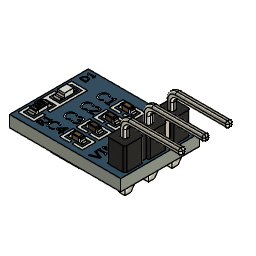
3V (Autodesk Fusion 360 design; units mm, degrees)
Autodesk Fusion 360 part; units mm, degrees
sketch "Sketch1" plane through (0, 0, 0) normal (0, 0, 1) x (1, 0, 0)
  line L0 (6, -4.25) -> (-6, -4.25)
  line L1 (-6, -4.25) -> (-6, 4.25)
  line L2 (-6, 4.25) -> (6, 4.25)
  line L3 (6, 4.25) -> (6, -4.25)
  line L4 (6, -4.25) -> (-6, 4.25) construction
  line L5 (-6, -4.25) -> (6, 4.25) construction
  dimension "d1" = 12
  dimension "d2" = 8.5
  constraint horizontal L0
  constraint perpendicular L0 L1
  constraint parallel L0 L2
  constraint parallel L1 L3
  constraint coincident L4 origin
  constraint coincident L5 origin
  measures "d1" distance of L1.end L2.end
  measures "d2" distance of L0.end L1.end
extrude "Extrude1" add sketch "Sketch1" along normal blind 1.25
sketch "Sketch2" plane through (0, 0, 1.25) normal (0, 0, 1) x (-1, 0, 0)
  line L0 (-6, -4.25) -> (6, -4.25)
  line L1 (6, -4.25) -> (6, 4.25)
  line L2 (6, 4.25) -> (-6, 4.25)
  line L3 (-6, 4.25) -> (-6, -4.25)
  line L4 (-5.75, 3.54) -> (-3.75, 3.54)
  line L5 (-3.75, 3.54) -> (-3.75, 1.54)
  line L6 (-3.75, 1.54) -> (-5.75, 1.54)
  line L7 (-5.75, 1.54) -> (-5.75, 3.54)
  line L8 (-5.75, 3.54) -> (-3.75, 1.54) construction
  line L9 (-3.75, 3.54) -> (-5.75, 1.54) construction
  line L10 (-5.075, 2.865) -> (-4.425, 2.865)
  line L11 (-4.425, 2.865) -> (-4.425, 2.215)
  line L12 (-4.425, 2.215) -> (-5.075, 2.215)
  line L13 (-5.075, 2.215) -> (-5.075, 2.865)
  line L14 (-5.075, 2.865) -> (-4.425, 2.215) construction
  line L15 (-4.425, 2.865) -> (-5.075, 2.215) construction
  line L16 (-5.5, 1.54) -> (-4, 1.54)
  line L17 (-4, 1.54) -> (-4, 1)
  line L18 (-4, 1) -> (-5.5, 1)
  line L19 (-5.5, 1) -> (-5.5, 1.54)
  line L20 (0.75, 2.65) -> (-0.75, 2.65)
  line L21 (-0.75, 2.65) -> (-0.75, 3.15)
  line L22 (-0.75, 3.15) -> (0.75, 3.15)
  line L23 (0.75, 3.15) -> (0.75, 2.65)
  line L24 (0.75, 2.65) -> (-0.75, 3.15) construction
  line L25 (-0.75, 2.65) -> (0.75, 3.15) construction
  line L26 (0.55, 3.15) -> (0.35, 3.15)
  line L27 (0.35, 3.15) -> (0.35, 2.65)
  line L28 (0.35, 2.65) -> (0.55, 2.65)
  line L29 (0.55, 2.65) -> (0.55, 3.15)
  line L30 (-0.35, 3.15) -> (-0.55, 3.15)
  line L31 (-0.55, 3.15) -> (-0.55, 2.65)
  line L32 (-0.55, 2.65) -> (-0.35, 2.65)
  line L33 (-0.35, 2.65) -> (-0.35, 3.15)
  line L34 (5.275, 3.1) -> (4.525, 3.1)
  line L35 (4.525, 3.1) -> (4.525, 1.1)
  line L36 (4.525, 1.1) -> (5.275, 1.1)
  line L37 (5.275, 1.1) -> (5.275, 3.1)
  line L38 (5.275, 3.1) -> (4.525, 1.1) construction
  line L39 (4.525, 3.1) -> (5.275, 1.1) construction
  line L40 (5.275, 1.35) -> (4.525, 1.35)
  line L41 (4.525, 1.35) -> (4.525, 1.6)
  line L42 (4.525, 1.6) -> (5.275, 1.6)
  line L43 (5.275, 1.6) -> (5.275, 1.35)
  line L44 (5.275, 2.6) -> (4.525, 2.6)
  line L45 (4.525, 2.6) -> (4.525, 2.85)
  line L46 (4.525, 2.85) -> (5.275, 2.85)
  line L47 (5.275, 2.85) -> (5.275, 2.6)
  line L48 (0.95, 2.45) -> (-0.95, 2.45)
  line L49 (-0.95, 2.45) -> (-0.95, 3.35)
  line L50 (-0.95, 3.35) -> (0.95, 3.35)
  line L51 (0.95, 3.35) -> (0.95, 2.45)
  line L52 (1.25, 2.15) -> (-1.25, 2.15)
  line L53 (-1.25, 2.15) -> (-1.25, 3.65)
  line L54 (-1.25, 3.65) -> (1.25, 3.65)
  line L55 (1.25, 3.65) -> (1.25, 2.15)
  line L56 (4.325, 0.9) -> (5.475, 0.9)
  line L57 (5.475, 0.9) -> (5.475, 3.3)
  line L58 (5.475, 3.3) -> (4.325, 3.3)
  line L59 (4.325, 3.3) -> (4.325, 0.9)
  line L60 (4.025, 0.6) -> (5.775, 0.6)
  line L61 (5.775, 0.6) -> (5.775, 3.6)
  line L62 (5.775, 3.6) -> (4.025, 3.6)
  line L63 (4.025, 3.6) -> (4.025, 0.6)
  line L64 (0.35, 2.65) -> (-0.35, 2.65)
  line L65 (-0.35, 2.65) -> (-0.35, 2.6501)
  line L66 (-0.35, 2.6501) -> (0.35, 2.6501)
  line L67 (0.35, 2.6501) -> (0.35, 2.65)
  line L68 (-0.35, 3.15) -> (0.35, 3.15)
  line L69 (0.35, 3.15) -> (0.35, 3.1499)
  line L70 (0.35, 3.1499) -> (-0.35, 3.1499)
  line L71 (-0.35, 3.1499) -> (-0.35, 3.15)
  line L72 (0.15, 3.35) -> (-0.15, 3.35)
  line L73 (-0.15, 3.35) -> (-0.15, 3.65)
  line L74 (-0.15, 3.65) -> (0.15, 3.65)
  line L75 (0.15, 3.65) -> (0.15, 3.35)
  line L76 (0.15, 3.35) -> (-0.15, 3.35)
  line L77 (-0.15, 3.35) -> (-0.15, 2.15)
  line L78 (-0.15, 2.15) -> (0.15, 2.15)
  line L79 (0.15, 2.15) -> (0.15, 3.35)
  line L80 (5.275, 2) -> (5.2749, 2)
  line L81 (5.2749, 1.6) -> (5.2749, 2.6)
  line L82 (5.2749, 3) -> (5.275, 3)
  line L83 (5.275, 2.6) -> (5.275, 1.6)
  line L84 (4.525, 1.6) -> (4.5251, 1.6)
  line L85 (4.5251, 1.6) -> (4.5251, 2.6)
  line L86 (4.5251, 2.6) -> (4.525, 2.6)
  line L87 (4.525, 2.6) -> (4.525, 1.6)
  line L88 (5.275, 2) -> (5.2749, 2)
  line L89 (5.2749, 1.6) -> (5.2749, 2.6)
  line L90 (5.2749, 2.6) -> (5.275, 2.6)
  line L91 (5.275, 2.6) -> (5.275, 1.6)
  line L92 (5.475, 1.85) -> (5.775, 1.85)
  line L93 (5.775, 1.85) -> (5.775, 2.35)
  line L94 (5.775, 2.35) -> (5.475, 2.35)
  line L95 (5.475, 2.35) -> (5.475, 1.85)
  line L96 (5.475, 1.85) -> (4.025, 1.85)
  line L97 (4.025, 1.85) -> (4.025, 2.35)
  line L98 (4.025, 2.35) -> (5.475, 2.35)
  line L99 (5.475, 2.35) -> (5.475, 1.85)
  line L100 (5.275, 0.3) -> (4.525, 0.3)
  line L101 (4.525, 0.3) -> (4.525, -1.7)
  line L102 (4.525, -1.7) -> (5.275, -1.7)
  line L103 (5.275, -1.7) -> (5.275, 0.3)
  line L104 (5.275, 0.3) -> (4.525, -1.7) construction
  line L105 (4.525, 0.3) -> (5.275, -1.7) construction
  line L106 (4.525, -1.7) -> (5.275, -1.7)
  line L107 (5.275, -1.7) -> (5.275, -1.2)
  line L108 (5.275, -1.2) -> (4.525, -1.2)
  line L109 (4.525, -1.2) -> (4.525, -1.7)
  line L110 (4.525, 0.3) -> (5.275, 0.3)
  line L111 (5.275, 0.3) -> (5.275, -0.2)
  line L112 (5.275, -0.2) -> (4.525, -0.2)
  line L113 (4.525, -0.2) -> (4.525, 0.3)
  line L114 (4.325, -1.9) -> (5.475, -1.9)
  line L115 (5.475, -1.9) -> (5.475, 0.5)
  line L116 (5.475, 0.5) -> (4.325, 0.5)
  line L117 (4.325, 0.5) -> (4.325, -1.9)
  line L118 (4.025, 0.8) -> (4.025, -2.2)
  line L119 (4.025, -2.2) -> (5.775, -2.2)
  line L120 (5.775, -2.2) -> (5.775, 0.8)
  line L121 (5.775, 0.8) -> (4.025, 0.8)
  line L122 (4.525, -0.2) -> (4.5251, -0.2)
  line L123 (4.5251, -0.2) -> (4.5251, -1.2)
  line L124 (4.5251, -1.2) -> (4.525, -1.2)
  line L125 (4.525, -1.2) -> (4.525, -0.2)
  line L126 (5.275, -0.2) -> (5.2749, -0.2)
  line L127 (5.2749, -0.2) -> (5.2749, -1.2)
  line L128 (5.2749, -1.2) -> (5.275, -1.2)
  line L129 (5.275, -1.2) -> (5.275, -0.2)
  line L130 (5.475, -0.35) -> (5.775, -0.35)
  line L131 (5.775, -0.35) -> (5.775, -0.85)
  line L132 (5.775, -0.85) -> (5.475, -0.85)
  line L133 (5.475, -0.85) -> (5.475, -0.35)
  line L134 (5.475, -0.85) -> (4.025, -0.85)
  line L135 (4.025, -0.85) -> (4.025, -0.35)
  line L136 (4.025, -0.35) -> (5.475, -0.35)
  line L137 (5.475, -0.35) -> (5.475, -0.85)
  point P0 (-4.75, 2.54)
  point P1 (-4.75, 2.54)
  point P2 (0, 2.9)
  point P3 (4.9, 2.1)
  point P4 (4.9, -0.7)
  dimension "d5" = 2
  dimension "d6" = 2
  dimension "d7" = 0.25
  dimension "d8" = 0.71
  dimension "d11" = 0.65
  dimension "d12" = 0.65
  dimension "d28" = 0.54
  dimension "d29" = 0.25
  dimension "d30" = 0.25
  dimension "d35" = 1.5
  dimension "d36" = 0.5
  dimension "d37" = 0.2
  dimension "d38" = 0.2
  dimension "d39" = 0.2
  dimension "d40" = 0.2
  dimension "d41" = 6
  dimension "d52" = 0.75
  dimension "d53" = 2
  dimension "d54" = 0.25
  dimension "d55" = 0.25
  dimension "d56" = 0.25
  dimension "d57" = 0.25
  dimension "d58" = 1.1
  dimension "d59" = 2.15
  dimension "d92" = -0.2
  dimension "d93" = -0.5
  dimension "d96" = 0.2
  dimension "d97" = 0.5
  dimension "d117" = 7.15
  dimension "d118" = 0.0001
  dimension "d119" = 0.0001
  dimension "d120" = 0.3
  dimension "d121" = 1.1
  dimension "d122" = 0.3
  dimension "d123" = 0.0001
  dimension "d124" = 0.0001
  dimension "d125" = 0.0001
  dimension "d128" = 0.5
  dimension "d129" = 1.25
  dimension "d130" = 0.5
  dimension "d131" = 0.75
  dimension "d132" = 2
  dimension "d133" = 1.1
  dimension "d134" = 3.55
  dimension "d135" = 0.5
  dimension "d136" = 0.5
  dimension "d137" = 0.2
  dimension "d138" = 0.5
  dimension "d143" = 0.0001
  dimension "d144" = 0.0001
  dimension "d147" = 0.5
  dimension "d148" = 0.95
  dimension "d149" = 0.5
  constraint horizontal L4
  constraint perpendicular L4 L5
  constraint parallel L4 L6
  constraint parallel L5 L7
  constraint coincident L8 P1
  constraint coincident L9 P1
  constraint horizontal L10
  constraint perpendicular L10 L11
  constraint parallel L10 L12
  constraint parallel L11 L13
  constraint coincident L14 P1
  constraint coincident L15 P1
  constraint coincident P1 P0
  constraint horizontal L16
  constraint vertical L17
  constraint horizontal L18
  constraint vertical L19
  constraint coincident L6 L16.start
  constraint horizontal L20
  constraint perpendicular L20 L21
  constraint parallel L20 L22
  constraint parallel L21 L23
  constraint coincident L24 P2
  constraint coincident L25 P2
  constraint horizontal L26
  constraint vertical L27
  constraint horizontal L28
  constraint vertical L29
  constraint coincident L22 L26.start
  constraint horizontal L30
  constraint vertical L31
  constraint horizontal L32
  constraint vertical L33
  constraint coincident L22 L30.start
  constraint horizontal L34
  constraint perpendicular L34 L35
  constraint parallel L34 L36
  constraint parallel L35 L37
  constraint coincident L38 P3
  constraint coincident L39 P3
  constraint horizontal L40
  constraint vertical L41
  constraint horizontal L42
  constraint vertical L43
  constraint coincident L37 L40.start
  constraint horizontal L44
  constraint vertical L45
  constraint horizontal L46
  constraint vertical L47
  constraint coincident L37 L44.start
  constraint coincident L20 L32.end
  constraint coincident L20 L27.end
  constraint coincident L35 L44.end
  constraint coincident L35 L41.end
  constraint horizontal L64
  constraint vertical L65
  constraint horizontal L66
  constraint vertical L67
  constraint coincident L33 L65.end
  constraint horizontal L68
  constraint vertical L69
  constraint horizontal L70
  constraint vertical L71
  constraint coincident L27 L69.end
  constraint horizontal L72
  constraint vertical L73
  constraint horizontal L74
  constraint vertical L75
  constraint coincident L54 L73.end
  constraint coincident L50 L72.start
  constraint horizontal L76
  constraint vertical L77
  constraint horizontal L78
  constraint vertical L79
  constraint coincident L52 L77.end
  constraint horizontal L80
  constraint vertical L81
  constraint horizontal L82
  constraint vertical L83
  constraint coincident L44 L81.end
  constraint horizontal L84
  constraint vertical L85
  constraint horizontal L86
  constraint vertical L87
  constraint coincident L44 L85.end
  constraint horizontal L88
  constraint vertical L89
  constraint horizontal L90
  constraint vertical L91
  constraint horizontal L92
  constraint vertical L93
  constraint horizontal L94
  constraint vertical L95
  constraint coincident L61 L93.end
  constraint coincident L57 L92.start
  constraint horizontal L96
  constraint vertical L97
  constraint horizontal L98
  constraint vertical L99
  constraint coincident L63 L97.end
  constraint horizontal L100
  constraint perpendicular L100 L101
  constraint parallel L100 L102
  constraint parallel L101 L103
  constraint coincident L104 P4
  constraint coincident L105 P4
  constraint horizontal L106
  constraint vertical L107
  constraint horizontal L108
  constraint vertical L109
  constraint coincident L103 L107.end
  constraint horizontal L110
  constraint vertical L111
  constraint horizontal L112
  constraint vertical L113
  constraint coincident L103 L111.end
  constraint horizontal L122
  constraint vertical L123
  constraint parallel L122 L124
  constraint vertical L125
  constraint horizontal L126
  constraint vertical L127
  constraint parallel L126 L128
  constraint vertical L129
  constraint coincident L108 L127.end
  constraint horizontal L130
  constraint vertical L131
  constraint horizontal L132
  constraint vertical L133
  constraint coincident L120 L131.end
  constraint coincident L115 L130.start
  constraint horizontal L134
  constraint vertical L135
  constraint horizontal L136
  constraint vertical L137
  constraint coincident L118 L135.end
  constraint coincident L108 L123.end
  measures "d5" distance of L5.end L6.end
  measures "d6" distance of L4.end L5.end
  measures "d7" distance of L3 L7
  measures "d8" distance of L2 L4
  measures "d11" distance of L11.end L12.end
  measures "d12" distance of L10.end L11.end
  measures "d28" distance of L16.start L18.end
  measures "d29" distance of L5 L17
  measures "d30" distance of L7 L19
  measures "d35" distance of L21.end L22.end
  measures "d36" distance of L20.end L21.end
  measures "d37" distance of L26.start L26.end
  measures "d38" distance of L30.start L30.end
  measures "d39" distance of L21 L31
  measures "d40" distance of L23 L29
  measures "d41" distance of L3 P2
  measures "d52" distance of L35.end L36.end
  measures "d53" distance of L34.end L35.end
  measures "d54" distance of L40.start L42.end
  measures "d55" distance of L36 L40
  measures "d56" distance of L44.start L46.end
  measures "d57" distance of L34 L46
  measures "d58" distance of L1 P3
  measures "d59" distance of L2 P3
  measures "d117" distance of L0 P2
  measures "d118" distance of L27.end L66.end
  measures "d119" distance of L30.start L70.end
  measures "d120" distance of L72.start L72.end
  measures "d121" distance of L53 L73
  measures "d122" distance of L72.start L72.end
  measures "d123" distance of L42.end L81.start
  measures "d124" distance of L41.end L84.end
  measures "d125" distance of L42.end L81.start
  measures "d128" distance of L92.start L94.end
  measures "d129" distance of L62 L94
  measures "d130" distance of L92.start L94.end
  measures "d131" distance of L101.end L102.end
  measures "d132" distance of L100.end L101.end
  measures "d133" distance of L1 P4
  measures "d134" distance of L0 P4
  measures "d135" distance of L101.end L108.end
  measures "d136" distance of L100.end L112.end
  measures "d143" distance of L112.end L122.end
  measures "d144" distance of L111.end L126.end
  measures "d147" distance of L130.start L132.end
  measures "d148" distance of L60 L130
  measures "d149" distance of L132.end L130.start
extrude "Extrude3" add sketch "Sketch2" along normal blind 4.5 contours L10 L11 L12 L13
extrude "Extrude2" add sketch "Sketch2" along normal blind 2.5 contours L4 L5 L6 L7 L16 | L10 L11 L12 L13
sketch "Sketch3" plane through (5.075, 0, 0) normal (1, 0, 0) x (0, 1, 0)
  line L0 (-2.865, 3.75) -> (-2.215, 3.75)
  line L1 (-2.215, 3.75) -> (-2.215, 5.75)
  line L2 (-2.215, 5.75) -> (-2.865, 5.75)
  line L3 (-2.865, 5.75) -> (-2.865, 3.75)
  line L4 (-2.865, 5.75) -> (-2.215, 5.75)
  line L5 (-2.215, 5.75) -> (-2.215, 5.1)
  line L6 (-2.215, 5.1) -> (-2.865, 5.1)
  line L7 (-2.865, 5.1) -> (-2.865, 5.75)
  dimension "d15" = 0.65
  constraint horizontal L4
  constraint vertical L5
  constraint horizontal L6
  constraint vertical L7
  constraint coincident L2.end L3.start
  constraint coincident L1 L5.end
  measures "d15" distance of L2.end L6.end
extrude "Extrude4" add sketch "Sketch3" along normal blind 6 contours L1 L2 L3 L4 L5 L6 L7
fillet "Fillet1" radius 0.2 16 edges at (5.075, -2.865, 4.425) (4.425, -2.865, 4.75) (5.075, -2.215, 4.425) (4.425, -2.215, 4.75) (7.75, -2.215, 5.75) (8.075, -2.215, 5.1) (7.75, -2.865, 5.75) (11.075, -2.54, 5.75) (11.075, -2.865, 5.425) (11.075, -2.215, 5.425) (11.075, -2.54, 5.1) (8.075, -2.865, 5.1) (5.75, -3.54, 2.5) (3.75, -3.54, 2.5) (5.75, -1.54, 2.5) (3.75, -1.54, 2.5)
fillet "Fillet1" radius 0.5 1 edges at (5.075, -2.54, 5.1)
fillet "Fillet1" radius 1 1 edges at (4.425, -2.54, 5.75)
pattern_linear "R-Pattern1" count 3 spacing 2.54 along (0, 1, 0) of "Extrude3", "Extrude2", "Extrude4", "Fillet1"
extrude "Extrude5" add sketch "Sketch2" along normal blind 2.5 contours L6 L16 L17 L18 L19
mirror "Mirror1" about plane through (0, 0, 0) normal (0, 1, 0) of "Extrude5"
extrude "Extrude6" add sketch "Sketch2" along normal blind 0.5 contours L20 L22 L26 L27 L28 L29 | L20 L22 L30 L31 L32 L33
extrude "Extrude7" add sketch "Sketch2" along normal blind 0.15 contours L20 L22 L23 L29 | L20 L21 L22 L31
extrude "Extrude8" add sketch "Sketch2" along normal blind 0.5001 contours L20 L22 L27 L64 L66 L68 L70 L79 | L20 L22 L64 L66 L68 L70 L77 L79 | L20 L22 L33 L64 L66 L68 L70 L77
fillet "Fillet2" radius 0.15 4 edges at (-0.55, -2.9, 1.4) (-0.75, -2.9, 1.4) (0.55, -2.9, 1.4) (0.75, -2.9, 1.4)
fillet "Fillet2" radius 0.05 8 edges at (0.45, -3.15, 1.75) (0, -3.1499, 1.7501) (-0.45, -3.15, 1.75) (-0.55, -2.9, 1.75) (-0.45, -2.65, 1.75) (0, -2.6501, 1.7501) (0.45, -2.65, 1.75) (0.55, -2.9, 1.75)
extrude "Extrude14" add sketch "Sketch2" along normal blind 0.001 contours L48 L50 L51 L52 L54 L55 L75 L79 | L48 L49 L50 L52 L53 L54 L73 L77
pattern_linear "R-Pattern2" count 4 spacing 1.8 along (0, 1, 0) of "Extrude6", "Extrude7", "Extrude8", "Fillet2", "Extrude14"
extrude "Extrude9" add sketch "Sketch2" along normal blind 0.4 contours L35 L37 L44 L45 L46 L47 | L35 L37 L40 L41 L42 L43
extrude "Extrude10" add sketch "Sketch2" along normal blind 0.15 contours L34 L35 L37 L46 | L35 L36 L37 L40
extrude "Extrude11" add sketch "Sketch2" along normal blind 0.4001 contours L35 L37 L44 L81 L83 L85 L87 L89 L91 L98 | L35 L37 L81 L83 L85 L87 L89 L91 L96 L98 | L35 L37 L42 L81 L83 L85 L87 L89 L91 L96
fillet "Fillet3" radius 0.15 4 edges at (-4.9, -2.85, 1.4) (-4.9, -3.1, 1.4) (-4.9, -1.35, 1.4) (-4.9, -1.1, 1.4)
fillet "Fillet3" radius 0.05 8 edges at (-4.9, -2.85, 1.65) (-5.275, -2.725, 1.65) (-5.2749, -2.1, 1.6501) (-5.275, -1.475, 1.65) (-4.9, -1.35, 1.65) (-4.525, -1.475, 1.65) (-4.5251, -2.1, 1.6501) (-4.525, -2.725, 1.65)
extrude "Extrude15" add sketch "Sketch2" along normal blind 0.001 contours L57 L58 L59 L61 L62 L63 L94 L98 | L56 L57 L59 L61 L63 L92 L96 L121 | L60 L61 L63 L118 L120 L121
extrude "Extrude19" add sketch "Sketch2" along normal blind 0.5 contours L101 L103 L112 L123 L125 L127 L129 L136 | L101 L103 L123 L125 L127 L129 L134 L136 | L101 L103 L108 L123 L125 L127 L129 L134
extrude "Extrude20" add sketch "Sketch2" along normal blind 0.15 contours L100 L101 L103 L110 L111 L112 L113 | L101 L102 L103 L106 L107 L108 L109
fillet "Fillet4" radius 0.15 4 edges at (-4.9, 1.2, 1.4) (-4.9, 1.7, 1.4) (-4.9, 0.2, 1.4) (-4.9, -0.3, 1.4)
extrude "Extrude21" add sketch "Sketch2" along normal blind 0.001 contours L60 L115 L116 L117 L118 L120 L130 L136 | L117 L118 L134 L135 L136 | L114 L115 L117 L118 L119 L120 L132 L134
sketch "Sketch4" plane through (0, 0, 0) normal (0, 0, -1) x (1, 0, 0)
  line L0 (-6, -4.25) -> (6, -4.25)
  line L1 (6, -4.25) -> (6, 4.25)
  line L2 (6, 4.25) -> (-6, 4.25)
  line L3 (-6, 4.25) -> (-6, -4.25)
  circle A0 centre (4.75, 2.54) radius 1
  line L4 (5.075, 2.215) -> (4.425, 2.215)
  line L5 (4.425, 2.215) -> (4.425, 2.865)
  line L6 (4.425, 2.865) -> (5.075, 2.865)
  line L7 (5.075, 2.865) -> (5.075, 2.215)
  line L8 (5.075, 2.215) -> (4.425, 2.865) construction
  line L9 (4.425, 2.215) -> (5.075, 2.865) construction
  point P0 (4.75, 2.54)
  point P1 (4.75, 2.54)
  dimension "d70" = 2
  dimension "d71" = 0.65
  dimension "d72" = 0.65
  constraint coincident P1 P0
  constraint horizontal L4
  constraint perpendicular L4 L5
  constraint parallel L4 L6
  constraint parallel L5 L7
  constraint coincident L8 P1
  constraint coincident L9 P1
  measures "d70" diameter of A0
  measures "d71" distance of L5.end L6.end
  measures "d72" distance of L4.end L5.end
extrude "Extrude12" add sketch "Sketch4" along normal blind 1.5 contours L4 L5 L6 L7
loft "Loft1" add profiles "Sketch4" section 1 contours A0 section 2 face at (4.8583, -2.4317, -1.5)
pattern_linear "R-Pattern4" count 3 spacing 2.54 along (0, 1, 0) of "Extrude12", "Loft1"
sketch "Sketch5" plane through (0, 0, 0) normal (0, 0, -1) x (1, 0, 0)
  spline S0 degree 3 poles (4.0429, -1.8329) (4.2258, -1.65) (4.4818, -1.5425) (4.7404, -1.54) (5.0054, -1.5375) (5.2697, -1.6455) (5.4571, -1.8329) knots -1 -1 -1 -1 -0.506107 -0.506107 -0.506107 0 0 0 0
  spline S1 degree 3 poles (5.4571, -1.8329) (5.64, -2.0158) (5.7475, -2.2718) (5.75, -2.5304) (5.7525, -2.7954) (5.6445, -3.0597) (5.4571, -3.2471) knots -1 -1 -1 -1 -0.506107 -0.506107 -0.506107 0 0 0 0
  spline S2 degree 3 poles (5.4571, -3.2471) (5.2742, -3.43) (5.0182, -3.5375) (4.7596, -3.54) (4.4946, -3.5425) (4.2303, -3.4345) (4.0429, -3.2471) knots -1 -1 -1 -1 -0.506107 -0.506107 -0.506107 0 0 0 0
  spline S3 degree 3 poles (4.0429, -3.2471) (3.86, -3.0642) (3.7525, -2.8082) (3.75, -2.5496) (3.7475, -2.2846) (3.8555, -2.0203) (4.0429, -1.8329) knots -1 -1 -1 -1 -0.506107 -0.506107 -0.506107 0 0 0 0
  spline S4 degree 3 poles (4.0429, 0.7071) (4.2258, 0.89) (4.4818, 0.9975) (4.7404, 1) (5.0054, 1.0025) (5.2697, 0.8945) (5.4571, 0.7071) knots -1 -1 -1 -1 -0.506107 -0.506107 -0.506107 0 0 0 0
  spline S5 degree 3 poles (5.4571, 0.7071) (5.64, 0.5242) (5.7475, 0.2682) (5.75, 0.0096) (5.7525, -0.2554) (5.6445, -0.5197) (5.4571, -0.7071) knots -1 -1 -1 -1 -0.506107 -0.506107 -0.506107 0 0 0 0
  spline S6 degree 3 poles (5.4571, -0.7071) (5.2742, -0.89) (5.0182, -0.9975) (4.7596, -1) (4.4946, -1.0025) (4.2303, -0.8945) (4.0429, -0.7071) knots -1 -1 -1 -1 -0.506107 -0.506107 -0.506107 0 0 0 0
  spline S7 degree 3 poles (4.0429, -0.7071) (3.86, -0.5242) (3.7525, -0.2682) (3.75, -0.0096) (3.7475, 0.2554) (3.8555, 0.5197) (4.0429, 0.7071) knots -1 -1 -1 -1 -0.506107 -0.506107 -0.506107 0 0 0 0
  spline S8 degree 3 poles (4.0429, 3.2471) (4.2258, 3.43) (4.4818, 3.5375) (4.7404, 3.54) (5.0054, 3.5425) (5.2697, 3.4345) (5.4571, 3.2471) knots -1 -1 -1 -1 -0.506107 -0.506107 -0.506107 0 0 0 0
  spline S9 degree 3 poles (5.4571, 3.2471) (5.64, 3.0642) (5.7475, 2.8082) (5.75, 2.5496) (5.7525, 2.2846) (5.6445, 2.0203) (5.4571, 1.8329) knots -1 -1 -1 -1 -0.506107 -0.506107 -0.506107 0 0 0 0
  spline S10 degree 3 poles (5.4571, 1.8329) (5.2742, 1.65) (5.0182, 1.5425) (4.7596, 1.54) (4.4946, 1.5375) (4.2303, 1.6455) (4.0429, 1.8329) knots -1 -1 -1 -1 -0.506107 -0.506107 -0.506107 0 0 0 0
  spline S11 degree 3 poles (4.0429, 1.8329) (3.86, 2.0158) (3.7525, 2.2718) (3.75, 2.5304) (3.7475, 2.7954) (3.8555, 3.0597) (4.0429, 3.2471) knots -1 -1 -1 -1 -0.506107 -0.506107 -0.506107 0 0 0 0
  line L0 (-6, -4.25) -> (6, -4.25)
  line L1 (6, -4.25) -> (6, 4.25)
  line L2 (6, 4.25) -> (-6, 4.25)
  line L3 (-6, 4.25) -> (-6, -4.25)
  line L4 (0.25, -3) -> (-3.25, -3)
  line L5 (-3.25, -3) -> (-3.25, 3)
  line L6 (-3.25, 3) -> (0.25, 3)
  line L7 (0.25, 3) -> (0.25, -3)
  line L8 (0.25, -3) -> (-3.25, 3) construction
  line L9 (-3.25, -3) -> (0.25, 3) construction
  point P0 (-1.5, 0)
  dimension "d152" = 3.5
  dimension "d153" = 6
  dimension "d154" = 4.5
  dimension "d155" = 4.25
  constraint horizontal L4
  constraint perpendicular L4 L5
  constraint parallel L4 L6
  constraint parallel L5 L7
  constraint coincident L8 P0
  constraint coincident L9 P0
  measures "d152" distance of L5.end L6.end
  measures "d153" distance of L4.end L5.end
  measures "d154" distance of L3 P0
  measures "d155" distance of L2 P0
extrude "Extrude22" add sketch "Sketch5" along normal blind 1.5 contours L4 L5 L6 L7
chamfer "Chamfer2" distance 0.2 distance2 0.9 1 faces at (-0.9167, 1, -1.5)
sketch "Sketch6" plane through (-3.25, 0, 0) normal (-1, 0, 0) x (0, -1, 0)
  line L0 (-3, -0.6) -> (3, -0.6)
  line L1 (3, -0.6) -> (3, 0)
  line L2 (3, 0) -> (-3, 0)
  line L3 (-3, 0) -> (-3, -0.6)
  line L4 (1.5, -0.6) -> (-1.5, -0.6)
  line L5 (-1.5, -0.6) -> (-1.5, -0.45)
  line L6 (-1.5, -0.45) -> (1.5, -0.45)
  line L7 (1.5, -0.45) -> (1.5, -0.6)
  dimension "d160" = 3
  dimension "d161" = 0.15
  dimension "d162" = 1.5
  constraint horizontal L4
  constraint vertical L5
  constraint horizontal L6
  constraint vertical L7
  constraint coincident L0 L4.start
  measures "d160" distance of L4.start L4.end
  measures "d161" distance of L4.start L6.end
  measures "d162" distance of L3 L5
extrude "Extrude23" add sketch "Sketch6" along normal blind 0.7 contours L0 L4 L5 L6 L7
sketch "Sketch7" plane through (0, 0, -0.6) normal (0, 0, -1) x (1, 0, 0)
  line L0 (-3.25, -1.5) -> (-3.25, 1.5)
  line L1 (-3.25, 1.5) -> (-3.95, 1.5)
  line L2 (-3.95, 1.5) -> (-3.95, -1.5)
  line L3 (-3.95, -1.5) -> (-3.25, -1.5)
  line L4 (-3.95, -1.5) -> (-3.8, -1.5)
  line L5 (-3.8, -1.5) -> (-3.8, 1.5)
  line L6 (-3.8, 1.5) -> (-3.95, 1.5)
  line L7 (-3.95, 1.5) -> (-3.95, -1.5)
  dimension "d165" = 0.15
  dimension "d166" = 3
  constraint horizontal L4
  constraint vertical L5
  constraint horizontal L6
  constraint vertical L7
  constraint coincident L2.end L3.start
  measures "d165" distance of L2.end L4.end
  measures "d166" distance of L2.end L1.end
extrude "Extrude24" add sketch "Sketch7" against normal blind 0.7 contours L1 L2 L3 L4 L5 L6 L7
sketch "Sketch8" plane through (-3.95, 0, 0) normal (-1, 0, 0) x (0, -1, 0)
  line L0 (-1.5, 0) -> (-1.5, -0.6)
  line L1 (-1.5, -0.6) -> (1.5, -0.6)
  line L2 (1.5, -0.6) -> (1.5, 0)
  line L3 (1.5, 0) -> (-1.5, 0)
  line L4 (1.5, 0) -> (-1.5, 0)
  line L5 (-1.5, 0) -> (-1.5, -0.15)
  line L6 (-1.5, -0.15) -> (1.5, -0.15)
  line L7 (1.5, -0.15) -> (1.5, 0)
  dimension "d169" = 0.15
  constraint horizontal L4
  constraint vertical L5
  constraint horizontal L6
  constraint vertical L7
  constraint coincident L0 L5.end
  constraint coincident L2.end L3.start
  measures "d169" distance of L2.end L6.end
extrude "Extrude25" add sketch "Sketch8" along normal blind 0.5 contours L0 L2 L3 L4 L5 L6 L7
fillet "Fillet5" radius 0.15 4 edges at (-3.95, 0, -0.6) (-3.95, 0, -0.15) (-4.45, 0, -0.15) (-3.8, 0, -0.45)
sketch "Sketch9" plane through (0, -1.5, 0) normal (0, -1, 0) x (1, 0, 0)
  arc A0 (-4.45, 0) -> (-4.3, -0.15) centre (-4.3, 0) ccw
  line L0 (-4.3, -0.15) -> (-4.1, -0.15)
  arc A1 (-3.95, -0.3) -> (-4.1, -0.15) centre (-4.1, -0.3) ccw
  line L1 (-3.95, -0.3) -> (-3.95, -0.45)
  arc A2 (-3.95, -0.45) -> (-3.8, -0.6) centre (-3.8, -0.45) ccw
  line L2 (-3.8, -0.6) -> (-3.25, -0.6)
  line L3 (-3.25, -0.6) -> (-3.25, -0.45)
  line L4 (-3.25, -0.45) -> (-3.65, -0.45)
  arc A3 (-3.8, -0.3) -> (-3.65, -0.45) centre (-3.65, -0.3) ccw
  line L5 (-3.8, -0.3) -> (-3.8, 0)
  line L6 (-3.8, 0) -> (-4.45, 0)
  line L7 (-4.45, 0) -> (-4.1, 0)
  arc A4 (-3.8, -0.3) -> (-4.1, 0) centre (-4.1, -0.3) ccw
  line L8 (-3.8, -0.3) -> (-3.8, -0.45)
  line L9 (-3.8, -0.45) -> (-3.25, -0.45)
  dimension "d174" = -0.15
  constraint coincident L3 L4.start
  constraint coincident A0.start L6.end
extrude "Extrude26" cut sketch "Sketch9" against normal blind 3 contours L5 L6 A4
sketch "Sketch10" plane through (0.25, 0, 0) normal (1, 0, 0) x (0, 1, 0)
  line L0 (-3, -0.6) -> (3, -0.6)
  line L1 (3, -0.6) -> (3, 0)
  line L2 (3, 0) -> (-3, 0)
  line L3 (-3, 0) -> (-3, -0.6)
  line L4 (2.75, -0.6) -> (1.75, -0.6)
  line L5 (1.75, -0.6) -> (1.75, -0.45)
  line L6 (1.75, -0.45) -> (2.75, -0.45)
  line L7 (2.75, -0.45) -> (2.75, -0.6)
  dimension "d177" = 1
  dimension "d178" = 0.15
  dimension "d179" = 0.25
  constraint horizontal L4
  constraint vertical L5
  constraint horizontal L6
  constraint vertical L7
  constraint coincident L0 L4.start
  measures "d177" distance of L4.start L4.end
  measures "d178" distance of L4.start L6.end
  measures "d179" distance of L1 L7
extrude "Extrude27" add sketch "Sketch10" along normal blind 0.7 contours L0 L4 L5 L6 L7
sketch "Sketch11" plane through (0, 0, -0.6) normal (0, 0, -1) x (1, 0, 0)
  line L0 (0.25, -1.75) -> (0.25, -2.75)
  line L1 (0.25, -2.75) -> (0.95, -2.75)
  line L2 (0.95, -2.75) -> (0.95, -1.75)
  line L3 (0.95, -1.75) -> (0.25, -1.75)
  line L4 (0.95, -1.75) -> (0.8, -1.75)
  line L5 (0.8, -1.75) -> (0.8, -2.75)
  line L6 (0.8, -2.75) -> (0.95, -2.75)
  line L7 (0.95, -2.75) -> (0.95, -1.75)
  dimension "d182" = 0.15
  constraint horizontal L4
  constraint vertical L5
  constraint horizontal L6
  constraint vertical L7
  constraint coincident L1 L5.end
  constraint coincident L2.end L3.start
  measures "d182" distance of L2.end L4.end
extrude "Extrude28" add sketch "Sketch11" against normal blind 0.7 contours L1 L2 L3 L4 L5 L6 L7
sketch "Sketch12" plane through (0.95, 0, 0) normal (1, 0, 0) x (0, 1, 0)
  line L0 (1.75, 0) -> (1.75, -0.6)
  line L1 (1.75, -0.6) -> (2.75, -0.6)
  line L2 (2.75, -0.6) -> (2.75, 0)
  line L3 (2.75, 0) -> (1.75, 0)
  line L4 (2.75, 0) -> (1.75, 0)
  line L5 (1.75, 0) -> (1.75, -0.15)
  line L6 (1.75, -0.15) -> (2.75, -0.15)
  line L7 (2.75, -0.15) -> (2.75, 0)
  dimension "d185" = 0.15
  constraint horizontal L4
  constraint vertical L5
  constraint horizontal L6
  constraint vertical L7
  constraint coincident L0 L5.end
  constraint coincident L2.end L3.start
  measures "d185" distance of L2.end L6.end
extrude "Extrude29" add sketch "Sketch12" along normal blind 0.5 contours L0 L2 L3 L4 L5 L6 L7
fillet "Fillet6" radius 0.15 4 edges at (0.95, 2.25, -0.6) (0.95, 2.25, -0.15) (1.45, 2.25, -0.15) (0.8, 2.25, -0.45)
sketch "Sketch13" plane through (0, 2.75, 0) normal (0, 1, 0) x (-1, 0, 0)
  arc A0 (-1.45, 0) -> (-1.3, -0.15) centre (-1.3, 0) ccw
  line L0 (-1.3, -0.15) -> (-1.1, -0.15)
  arc A1 (-0.95, -0.3) -> (-1.1, -0.15) centre (-1.1, -0.3) ccw
  line L1 (-0.95, -0.3) -> (-0.95, -0.45)
  arc A2 (-0.95, -0.45) -> (-0.8, -0.6) centre (-0.8, -0.45) ccw
  line L2 (-0.8, -0.6) -> (-0.25, -0.6)
  line L3 (-0.25, -0.6) -> (-0.25, -0.45)
  line L4 (-0.25, -0.45) -> (-0.65, -0.45)
  arc A3 (-0.8, -0.3) -> (-0.65, -0.45) centre (-0.65, -0.3) ccw
  line L5 (-0.8, -0.3) -> (-0.8, 0)
  line L6 (-0.8, 0) -> (-1.45, 0)
  line L7 (-1.45, 0) -> (-1.1, 0)
  arc A4 (-0.8, -0.3) -> (-1.1, 0) centre (-1.1, -0.3) ccw
  line L8 (-0.8, -0.3) -> (-0.8, -0.45)
  line L9 (-0.8, -0.45) -> (-0.25, -0.45)
  dimension "d190" = -0.15
  constraint coincident A0.start L6.end
  constraint coincident L3 L4.start
extrude "Extrude30" cut sketch "Sketch13" against normal blind 1 contours L5 L6 A4
pattern_linear "R-Pattern5" count 3 spacing 2.25 along (0, -1, 0) of "Extrude27", "Extrude28", "Extrude29", "Fillet6", "Extrude30"
sketch "Sketch14" plane through (0, 0, 1.25) normal (0, 0, 1) x (-1, 0, 0)
  line L0 (-6, -4.25) -> (6, -4.25)
  line L1 (6, -4.25) -> (6, 4.25)
  line L2 (6, 4.25) -> (-6, 4.25)
  line L3 (-6, 4.25) -> (-6, -4.25)
  line L4 (-5.5, -1.54) -> (-5.5, -1)
  line L5 (-5.5, -1) -> (-5.55, -1)
  arc A0 (-5.75, -0.8) -> (-5.55, -1) centre (-5.55, -0.8) ccw
  line L6 (-5.75, -0.8) -> (-5.75, 0.8)
  arc A1 (-5.55, 1) -> (-5.75, 0.8) centre (-5.55, 0.8) ccw
  line L7 (-5.55, 1) -> (-5.5, 1)
  line L8 (-5.5, 1) -> (-5.5, 1.54)
  line L9 (-5.5, 1.54) -> (-5.55, 1.54)
  arc A2 (-5.75, 1.74) -> (-5.55, 1.54) centre (-5.55, 1.74) ccw
  line L10 (-5.75, 1.74) -> (-5.75, 3.34)
  arc A3 (-5.55, 3.54) -> (-5.75, 3.34) centre (-5.55, 3.34) ccw
  line L11 (-5.55, 3.54) -> (-3.95, 3.54)
  arc A4 (-3.75, 3.34) -> (-3.95, 3.54) centre (-3.95, 3.34) ccw
  line L12 (-3.75, 3.34) -> (-3.75, 1.74)
  arc A5 (-3.95, 1.54) -> (-3.75, 1.74) centre (-3.95, 1.74) ccw
  line L13 (-3.95, 1.54) -> (-4, 1.54)
  line L14 (-4, 1.54) -> (-4, 1)
  line L15 (-4, 1) -> (-3.95, 1)
  arc A6 (-3.75, 0.8) -> (-3.95, 1) centre (-3.95, 0.8) ccw
  line L16 (-3.75, 0.8) -> (-3.75, -0.8)
  arc A7 (-3.95, -1) -> (-3.75, -0.8) centre (-3.95, -0.8) ccw
  line L17 (-3.95, -1) -> (-4, -1)
  line L18 (-4, -1) -> (-4, -1.54)
  line L19 (-4, -1.54) -> (-3.95, -1.54)
  arc A8 (-3.75, -1.74) -> (-3.95, -1.54) centre (-3.95, -1.74) ccw
  line L20 (-3.75, -1.74) -> (-3.75, -3.34)
  arc A9 (-3.95, -3.54) -> (-3.75, -3.34) centre (-3.95, -3.34) ccw
  line L21 (-3.95, -3.54) -> (-5.55, -3.54)
  arc A10 (-5.75, -3.34) -> (-5.55, -3.54) centre (-5.55, -3.34) ccw
  line L22 (-5.75, -3.34) -> (-5.75, -1.74)
  arc A11 (-5.55, -1.54) -> (-5.75, -1.74) centre (-5.55, -1.74) ccw
  line L23 (-5.55, -1.54) -> (-5.5, -1.54)
  line L24 (1.25, 3.65) -> (1.25, 2.15)
  line L25 (-0.15, 2.15) -> (-1.25, 2.15)
  line L26 (-1.25, 2.15) -> (-1.25, 3.65)
  line L27 (-1.25, 3.65) -> (-0.15, 3.65)
  line L28 (1.25, 1.85) -> (1.25, 0.35)
  line L29 (1.25, 0.35) -> (0.15, 0.35)
  line L30 (-1.25, 0.35) -> (-1.25, 1.85)
  line L31 (0.15, 1.85) -> (1.25, 1.85)
  line L32 (1.25, 0.05) -> (1.25, -1.45)
  line L33 (-0.15, -1.45) -> (-1.25, -1.45)
  line L34 (-1.25, -1.45) -> (-1.25, 0.05)
  line L35 (-1.25, 0.05) -> (-0.15, 0.05)
  line L36 (1.25, -1.75) -> (1.25, -3.25)
  line L37 (1.25, -3.25) -> (0.15, -3.25)
  line L38 (-1.25, -3.25) -> (-1.25, -1.75)
  line L39 (0.15, -1.75) -> (1.25, -1.75)
  line L40 (4.025, 3.6) -> (5.775, 3.6)
  line L41 (5.775, 1.85) -> (5.775, -0.35)
  line L42 (4.025, -2.2) -> (4.025, 1.85)
  line L43 (3.1789, -1.7897) -> (1.3303, -1.7897) construction
  line L44 (1.3303, -1.7897) -> (1.3303, -3.1651) construction
  line L45 (1.3303, -3.1651) -> (3.1789, -3.1651) construction
  line L46 (3.1789, -3.1651) -> (3.1789, -1.7897) construction
  line L47 (3.1855, -0.0301) -> (1.3369, -0.0301) construction
  line L48 (1.3369, -0.0301) -> (1.3369, -1.4054) construction
  line L49 (1.3369, -1.4054) -> (3.1855, -1.4054) construction
  line L50 (3.1855, -1.4054) -> (3.1855, -0.0301) construction
  line L51 (3.1525, 3.5727) -> (1.3038, 3.5727) construction
  line L52 (1.3038, 3.5727) -> (1.3038, 2.1974) construction
  line L53 (1.3038, 2.1974) -> (3.1525, 2.1974) construction
  line L54 (3.1525, 2.1974) -> (3.1525, 3.5727) construction
  line L55 (3.1627, 1.7821) -> (1.3141, 1.7821) construction
  line L56 (1.3141, 1.7821) -> (1.3141, 0.4068) construction
  line L57 (1.3141, 0.4068) -> (3.1627, 0.4068) construction
  line L58 (3.1627, 0.4068) -> (3.1627, 1.7821) construction
  line L59 (-3.209, 3.6614) -> (-3.209, 1.8128) construction
  line L60 (-3.209, 1.8128) -> (-1.8337, 1.8128) construction
  line L61 (-1.8337, 1.8128) -> (-1.8337, 3.6614) construction
  line L62 (-1.8337, 3.6614) -> (-3.209, 3.6614) construction
  line L63 (-3.209, 1.0614) -> (-3.209, -0.7872) construction
  line L64 (-3.209, -0.7872) -> (-1.8337, -0.7872) construction
  line L65 (-1.8337, -0.7872) -> (-1.8337, 1.0614) construction
  line L66 (-1.8337, 1.0614) -> (-3.209, 1.0614) construction
  line L67 (-3.209, -1.6886) -> (-3.209, -3.5372) construction
  line L68 (-3.209, -3.5372) -> (-1.8337, -3.5372) construction
  line L69 (-1.8337, -3.5372) -> (-1.8337, -1.6886) construction
  line L70 (-1.8337, -1.6886) -> (-3.209, -1.6886) construction
  line L71 (2.8382, 3.8814) -> (2.8382, 2.0328) construction
  line L72 (2.8382, 2.0328) -> (4.2136, 2.0328) construction
  line L73 (4.2136, 2.0328) -> (4.2136, 3.8814) construction
  line L74 (4.2136, 3.8814) -> (2.8382, 3.8814) construction
  line L75 (4.5641, -2.5206) -> (4.5641, -4.3692) construction
  line L76 (4.5641, -4.3692) -> (5.9395, -4.3692) construction
  line L77 (5.9395, -4.3692) -> (5.9395, -2.5206) construction
  line L78 (5.9395, -2.5206) -> (4.5641, -2.5206) construction
  line L79 (4.025, 1.85) -> (4.325, 1.85)
  line L80 (4.325, 1.85) -> (4.325, 0.9)
  line L81 (4.325, 0.9) -> (5.475, 0.9)
  line L82 (5.475, 0.9) -> (5.475, 1.85)
  line L83 (5.475, 1.85) -> (5.775, 1.85)
  line L84 (5.775, -0.35) -> (5.475, -0.35)
  line L85 (5.475, -0.35) -> (5.475, 0.5)
  line L86 (5.475, 0.5) -> (4.325, 0.5)
  line L87 (4.325, 0.5) -> (4.325, -1.9)
  line L88 (4.325, -1.9) -> (5.475, -1.9)
  line L89 (5.475, -1.9) -> (5.475, -0.85)
  line L90 (5.475, -0.85) -> (5.775, -0.85)
  line L91 (5.775, -0.85) -> (5.775, -2.2)
  line L92 (5.775, -2.2) -> (4.025, -2.2)
  line L93 (0.15, -3.25) -> (0.15, -2.95)
  line L94 (0.15, -2.95) -> (0.95, -2.95)
  line L95 (0.95, -2.95) -> (0.95, -2.05)
  line L96 (0.95, -2.05) -> (0.15, -2.05)
  line L97 (0.15, -2.05) -> (0.15, -1.75)
  line L98 (-0.15, -3.25) -> (-1.25, -3.25)
  line L99 (-1.25, -1.75) -> (-0.15, -1.75)
  line L100 (-0.15, -1.75) -> (-0.15, -2.05)
  line L101 (-0.15, -2.05) -> (-0.95, -2.05)
  line L102 (-0.95, -2.05) -> (-0.95, -2.95)
  line L103 (-0.95, -2.95) -> (-0.15, -2.95)
  line L104 (-0.15, -2.95) -> (-0.15, -3.25)
  line L105 (0.35, -0.9499) -> (-0.35, -0.9499)
  line L106 (-0.35, -0.9499) -> (-0.35, -0.95)
  line L107 (-0.35, -0.95) -> (-0.75, -0.95)
  line L108 (-0.75, -0.95) -> (-0.75, -0.45)
  line L109 (-0.75, -0.45) -> (-0.35, -0.45)
  line L110 (-0.35, -0.45) -> (-0.35, -0.4501)
  line L111 (-0.35, -0.4501) -> (0.35, -0.4501)
  line L112 (0.35, -0.4501) -> (0.35, -0.45)
  line L113 (0.35, -0.45) -> (0.75, -0.45)
  line L114 (0.75, -0.45) -> (0.75, -0.95)
  line L115 (0.75, -0.95) -> (0.35, -0.95)
  line L116 (0.35, -0.95) -> (0.35, -0.9499)
  line L117 (0.15, 0.35) -> (0.15, 0.65)
  line L118 (0.15, 0.65) -> (0.95, 0.65)
  line L119 (0.95, 0.65) -> (0.95, 1.55)
  line L120 (0.95, 1.55) -> (0.15, 1.55)
  line L121 (0.15, 1.55) -> (0.15, 1.85)
  line L122 (-0.15, 0.35) -> (-1.25, 0.35)
  line L123 (-1.25, 1.85) -> (-0.15, 1.85)
  line L124 (-0.15, 1.85) -> (-0.15, 1.55)
  line L125 (-0.15, 1.55) -> (-0.95, 1.55)
  line L126 (-0.95, 1.55) -> (-0.95, 0.65)
  line L127 (-0.95, 0.65) -> (-0.15, 0.65)
  line L128 (-0.15, 0.65) -> (-0.15, 0.35)
  line L129 (0.35, 2.6501) -> (-0.35, 2.6501)
  line L130 (-0.35, 2.6501) -> (-0.35, 2.65)
  line L131 (-0.35, 2.65) -> (-0.75, 2.65)
  line L132 (-0.75, 2.65) -> (-0.75, 3.15)
  line L133 (-0.75, 3.15) -> (-0.35, 3.15)
  line L134 (-0.35, 3.15) -> (-0.35, 3.1499)
  line L135 (-0.35, 3.1499) -> (0.35, 3.1499)
  line L136 (0.35, 3.1499) -> (0.35, 3.15)
  line L137 (0.35, 3.15) -> (0.75, 3.15)
  line L138 (0.75, 3.15) -> (0.75, 2.65)
  line L139 (0.75, 2.65) -> (0.35, 2.65)
  line L140 (0.35, 2.65) -> (0.35, 2.6501)
  line L141 (-0.15, 3.65) -> (-0.15, 3.35)
  line L142 (-0.15, 3.35) -> (-0.95, 3.35)
  line L143 (-0.95, 3.35) -> (-0.95, 2.45)
  line L144 (-0.95, 2.45) -> (-0.15, 2.45)
  line L145 (-0.15, 2.45) -> (-0.15, 2.15)
  line L146 (0.15, 3.65) -> (1.25, 3.65)
  line L147 (1.25, 2.15) -> (0.15, 2.15)
  line L148 (0.15, 2.15) -> (0.15, 2.45)
  line L149 (0.15, 2.45) -> (0.95, 2.45)
  line L150 (0.95, 2.45) -> (0.95, 3.35)
  line L151 (0.95, 3.35) -> (0.15, 3.35)
  line L152 (0.15, 3.35) -> (0.15, 3.65)
  line L153 (0.35, 0.8501) -> (-0.35, 0.8501)
  line L154 (-0.35, 0.8501) -> (-0.35, 0.85)
  line L155 (-0.35, 0.85) -> (-0.75, 0.85)
  line L156 (-0.75, 0.85) -> (-0.75, 1.35)
  line L157 (-0.75, 1.35) -> (-0.35, 1.35)
  line L158 (-0.35, 1.35) -> (-0.35, 1.3499)
  line L159 (-0.35, 1.3499) -> (0.35, 1.3499)
  line L160 (0.35, 1.3499) -> (0.35, 1.35)
  line L161 (0.35, 1.35) -> (0.75, 1.35)
  line L162 (0.75, 1.35) -> (0.75, 0.85)
  line L163 (0.75, 0.85) -> (0.35, 0.85)
  line L164 (0.35, 0.85) -> (0.35, 0.8501)
  line L165 (-0.15, 0.05) -> (-0.15, -0.25)
  line L166 (-0.15, -0.25) -> (-0.95, -0.25)
  line L167 (-0.95, -0.25) -> (-0.95, -1.15)
  line L168 (-0.95, -1.15) -> (-0.15, -1.15)
  line L169 (-0.15, -1.15) -> (-0.15, -1.45)
  line L170 (0.15, 0.05) -> (1.25, 0.05)
  line L171 (1.25, -1.45) -> (0.15, -1.45)
  line L172 (0.15, -1.45) -> (0.15, -1.15)
  line L173 (0.15, -1.15) -> (0.95, -1.15)
  line L174 (0.95, -1.15) -> (0.95, -0.25)
  line L175 (0.95, -0.25) -> (0.15, -0.25)
  line L176 (0.15, -0.25) -> (0.15, 0.05)
  line L177 (0.35, -2.7499) -> (-0.35, -2.7499)
  line L178 (-0.35, -2.7499) -> (-0.35, -2.75)
  line L179 (-0.35, -2.75) -> (-0.75, -2.75)
  line L180 (-0.75, -2.75) -> (-0.75, -2.25)
  line L181 (-0.75, -2.25) -> (-0.35, -2.25)
  line L182 (-0.35, -2.25) -> (-0.35, -2.2501)
  line L183 (-0.35, -2.2501) -> (0.35, -2.2501)
  line L184 (0.35, -2.2501) -> (0.35, -2.25)
  line L185 (0.35, -2.25) -> (0.75, -2.25)
  line L186 (0.75, -2.25) -> (0.75, -2.75)
  line L187 (0.75, -2.75) -> (0.35, -2.75)
  line L188 (0.35, -2.75) -> (0.35, -2.7499)
  line L189 (5.2749, 2.6) -> (5.2749, 1.6)
  line L190 (5.2749, 1.6) -> (5.275, 1.6)
  line L191 (5.275, 1.6) -> (5.275, 1.1)
  line L192 (5.275, 1.1) -> (4.525, 1.1)
  line L193 (4.525, 1.1) -> (4.525, 1.6)
  line L194 (4.525, 1.6) -> (4.5251, 1.6)
  line L195 (4.5251, 1.6) -> (4.5251, 2.6)
  line L196 (4.5251, 2.6) -> (4.525, 2.6)
  line L197 (4.525, 2.6) -> (4.525, 3.1)
  line L198 (4.525, 3.1) -> (5.275, 3.1)
  line L199 (5.275, 3.1) -> (5.275, 2.6)
  line L200 (5.275, 2.6) -> (5.2749, 2.6)
  line L201 (5.475, 2.35) -> (5.475, 3.3)
  line L202 (5.475, 3.3) -> (4.325, 3.3)
  line L203 (4.325, 3.3) -> (4.325, 2.35)
  line L204 (4.325, 2.35) -> (4.025, 2.35)
  line L205 (4.025, 2.35) -> (4.025, 3.6)
  line L206 (5.775, 3.6) -> (5.775, 2.35)
  line L207 (5.775, 2.35) -> (5.475, 2.35)
  line L208 (5.2749, -1.2) -> (5.275, -1.2)
  line L209 (5.275, -1.2) -> (5.275, -1.7)
  line L210 (5.275, -1.7) -> (4.525, -1.7)
  line L211 (4.525, -1.7) -> (4.525, -1.2)
  line L212 (4.525, -1.2) -> (4.5251, -1.2)
  line L213 (4.5251, -1.2) -> (4.5251, -0.2)
  line L214 (4.5251, -0.2) -> (4.525, -0.2)
  line L215 (4.525, -0.2) -> (4.525, 0.3)
  line L216 (4.525, 0.3) -> (5.275, 0.3)
  line L217 (5.275, 0.3) -> (5.275, -0.2)
  line L218 (5.275, -0.2) -> (5.2749, -0.2)
  line L219 (5.2749, -0.2) -> (5.2749, -1.2)
  dimension "d100" = 1
  dimension "d101" = 1
  dimension "d102" = 1
  dimension "d103" = 1
  dimension "d104" = 0.9
  dimension "d105" = 0.9
  dimension "d106" = 0.9
  dimension "d107" = 0.7
  dimension "d108" = 0.7
  text T0 "C1" font "Verdana" height 1 align centre middle in box 1.8486 x 1.3754 at (3.1789, -1.7897) x (-1, 0) y (0, -1) spacing 1 kerned
  text T1 "C2" font "Verdana" height 1 align centre middle in box 1.8486 x 1.3754 at (3.1855, -0.0301) x (-1, 0) y (0, -1) spacing 1 kerned
  text T2 "C4" font "Verdana" height 1 align centre middle in box 1.8486 x 1.3754 at (3.1525, 3.5727) x (-1, 0) y (0, -1) spacing 1 kerned
  text T3 "C3" font "Verdana" height 1 align centre middle in box 1.8486 x 1.3754 at (3.1627, 1.7821) x (-1, 0) y (0, -1) spacing 1 kerned
  text T4 "VIN" font "Verdana" height 0.9 align centre middle in box 1.8486 x 1.3754 at (-3.209, 3.6614) x (0, -1) y (1, 0) spacing 1 kerned
  text T5 "OUT" font "Verdana" height 0.9 align centre middle in box 1.8486 x 1.3754 at (-3.209, 1.0614) x (0, -1) y (1, 0) spacing 1 kerned
  text T6 "GND" font "Verdana" height 0.9 align centre middle in box 1.8486 x 1.3754 at (-3.209, -1.6886) x (0, -1) y (1, 0) spacing 1 kerned
  text T7 "R1" font "Verdana" height 0.7 align centre middle in box 1.8486 x 1.3754 at (2.8382, 3.8814) x (0, -1) y (1, 0) spacing 1 kerned
  text T8 "D1" font "Verdana" height 0.7 align centre middle in box 1.8486 x 1.3754 at (4.5641, -2.5206) x (0, -1) y (1, 0) spacing 1 kerned
extrude "Extrude16" add sketch "Sketch14" along normal blind 0.001 text T7 T8 T0 T1 T3 T2 T4 T5 T6
sketch "Sketch15" plane through (0, 0, 1.6501) normal (0, 0, 1) x (-1, 0, 0)
  line L0 (4.5751, 1.6) -> (5.2249, 1.6)
  line L1 (5.2249, 2.6) -> (4.5751, 2.6)
  line L2 (5.2249, 1.6) -> (5.2249, 2.6) construction
  line L3 (5.2249, 2.6) -> (4.5751, 2.6) construction
  line L4 (4.5751, 2.6) -> (4.5751, 1.6) construction
  line L5 (4.5751, 1.6) -> (5.2249, 1.6) construction
  line L6 (4.5751, 2.6) -> (4.5751, 1.6)
  line L7 (5.2249, 1.6) -> (5.2249, 2.6)
  dimension "d111" = 0.35
  text T0 "102" font "Verdana" height 0.35 align centre middle in box 1 x 0.6498 at (5.2249, 1.6) x (0, 1) y (-1, 0) spacing 1 kerned mirrored across
  constraint coincident L0.start
  constraint coincident L1.start
extrude "Extrude17" add sketch "Sketch15" along normal blind 0.001 text T0
sketch "Sketch16" plane through (0, 0, 0) normal (0, 0, -1) x (1, 0, 0)
  spline S0 degree 3 poles (4.0429, -1.8329) (4.2258, -1.65) (4.4818, -1.5425) (4.7404, -1.54) (5.0054, -1.5375) (5.2697, -1.6455) (5.4571, -1.8329) knots -1 -1 -1 -1 -0.506107 -0.506107 -0.506107 0 0 0 0
  spline S1 degree 3 poles (5.4571, -1.8329) (5.64, -2.0158) (5.7475, -2.2718) (5.75, -2.5304) (5.7525, -2.7954) (5.6445, -3.0597) (5.4571, -3.2471) knots -1 -1 -1 -1 -0.506107 -0.506107 -0.506107 0 0 0 0
  spline S2 degree 3 poles (5.4571, -3.2471) (5.2742, -3.43) (5.0182, -3.5375) (4.7596, -3.54) (4.4946, -3.5425) (4.2303, -3.4345) (4.0429, -3.2471) knots -1 -1 -1 -1 -0.506107 -0.506107 -0.506107 0 0 0 0
  spline S3 degree 3 poles (4.0429, -3.2471) (3.86, -3.0642) (3.7525, -2.8082) (3.75, -2.5496) (3.7475, -2.2846) (3.8555, -2.0203) (4.0429, -1.8329) knots -1 -1 -1 -1 -0.506107 -0.506107 -0.506107 0 0 0 0
  spline S4 degree 3 poles (4.0429, 0.7071) (4.2258, 0.89) (4.4818, 0.9975) (4.7404, 1) (5.0054, 1.0025) (5.2697, 0.8945) (5.4571, 0.7071) knots -1 -1 -1 -1 -0.506107 -0.506107 -0.506107 0 0 0 0
  spline S5 degree 3 poles (5.4571, 0.7071) (5.64, 0.5242) (5.7475, 0.2682) (5.75, 0.0096) (5.7525, -0.2554) (5.6445, -0.5197) (5.4571, -0.7071) knots -1 -1 -1 -1 -0.506107 -0.506107 -0.506107 0 0 0 0
  spline S6 degree 3 poles (5.4571, -0.7071) (5.2742, -0.89) (5.0182, -0.9975) (4.7596, -1) (4.4946, -1.0025) (4.2303, -0.8945) (4.0429, -0.7071) knots -1 -1 -1 -1 -0.506107 -0.506107 -0.506107 0 0 0 0
  spline S7 degree 3 poles (4.0429, -0.7071) (3.86, -0.5242) (3.7525, -0.2682) (3.75, -0.0096) (3.7475, 0.2554) (3.8555, 0.5197) (4.0429, 0.7071) knots -1 -1 -1 -1 -0.506107 -0.506107 -0.506107 0 0 0 0
  spline S8 degree 3 poles (4.0429, 3.2471) (4.2258, 3.43) (4.4818, 3.5375) (4.7404, 3.54) (5.0054, 3.5425) (5.2697, 3.4345) (5.4571, 3.2471) knots -1 -1 -1 -1 -0.506107 -0.506107 -0.506107 0 0 0 0
  spline S9 degree 3 poles (5.4571, 3.2471) (5.64, 3.0642) (5.7475, 2.8082) (5.75, 2.5496) (5.7525, 2.2846) (5.6445, 2.0203) (5.4571, 1.8329) knots -1 -1 -1 -1 -0.506107 -0.506107 -0.506107 0 0 0 0
  spline S10 degree 3 poles (5.4571, 1.8329) (5.2742, 1.65) (5.0182, 1.5425) (4.7596, 1.54) (4.4946, 1.5375) (4.2303, 1.6455) (4.0429, 1.8329) knots -1 -1 -1 -1 -0.506107 -0.506107 -0.506107 0 0 0 0
  spline S11 degree 3 poles (4.0429, 1.8329) (3.86, 2.0158) (3.7525, 2.2718) (3.75, 2.5304) (3.7475, 2.7954) (3.8555, 3.0597) (4.0429, 3.2471) knots -1 -1 -1 -1 -0.506107 -0.506107 -0.506107 0 0 0 0
  line L0 (-6, -4.25) -> (6, -4.25)
  line L1 (6, -4.25) -> (6, 4.25)
  line L2 (6, 4.25) -> (-6, 4.25)
  line L3 (-6, 4.25) -> (-6, -4.25)
  line L4 (-4.574, -4.1846) -> (-4.574, -2.2846) construction
  line L5 (-4.574, -2.2846) -> (-5.874, -2.2846) construction
  line L6 (-5.874, -2.2846) -> (-5.874, -4.1846) construction
  line L7 (-5.874, -4.1846) -> (-4.574, -4.1846) construction
  line L8 (1.1, 0.5) -> (1.45, 0.5)
  line L9 (1.45, 0.5) -> (1.45, -0.5)
  line L10 (1.45, -0.5) -> (1.1, -0.5)
  line L11 (1.1, -0.5) -> (1.1, 0.5)
  line L12 (-4.1, -1.5) -> (-4.45, -1.5)
  line L13 (-4.45, -1.5) -> (-4.45, 1.5)
  line L14 (-4.45, 1.5) -> (-4.1, 1.5)
  line L15 (-4.1, 1.5) -> (-4.1, -1.5)
  line L16 (0.25, 3) -> (0.25, -3)
  line L17 (0.25, -3) -> (-3.25, -3)
  line L18 (-3.25, -3) -> (-3.25, 3)
  line L19 (-3.25, 3) -> (0.25, 3)
  line L20 (1.1, -1.75) -> (1.45, -1.75)
  line L21 (1.45, -1.75) -> (1.45, -2.75)
  line L22 (1.45, -2.75) -> (1.1, -2.75)
  line L23 (1.1, -2.75) -> (1.1, -1.75)
  line L24 (1.1, 2.75) -> (1.45, 2.75)
  line L25 (1.45, 2.75) -> (1.45, 1.75)
  line L26 (1.45, 1.75) -> (1.1, 1.75)
  line L27 (1.1, 1.75) -> (1.1, 2.75)
  line L28 (-3.55, 3.3) -> (0.55, 3.3)
  line L29 (0.55, 3.3) -> (0.55, -3.3)
  line L30 (0.55, -3.3) -> (-3.55, -3.3)
  line L31 (-3.55, -3.3) -> (-3.55, 3.3)
  dimension "d114" = 0.75
  dimension "d197" = -0.3
  text T0 "U1" font "Verdana" height 0.75 align centre middle in box 1.9 x 1.3 at (-4.574, -4.1846) x (0, 1) y (-1, 0) spacing 1 kerned
extrude "Extrude18" add sketch "Sketch16" sketch "Sketch16" along normal blind 0.001 contours L28 L29 L30 L31 of sketch 2 text T0
sketch "Sketch17" plane through (0, 0, -1.5) normal (0, 0, -1) x (1, 0, 0)
  line L0 (-3.05, -2.8) -> (0.05, -2.8)
  line L1 (0.05, -2.8) -> (0.05, 2.8)
  line L2 (0.05, 2.8) -> (-3.05, 2.8)
  line L3 (-3.05, 2.8) -> (-3.05, -2.8)
  line L4 (0.05, -2.8) -> (0.05, 2.8) construction
  line L5 (0.05, 2.8) -> (-3.05, 2.8) construction
  line L6 (-3.05, 2.8) -> (-3.05, -2.8) construction
  line L7 (-3.05, -2.8) -> (0.05, -2.8) construction
  dimension "d198" = 0.7
  text T0 "AMS1117\n33  D203" font "Verdana" height 0.7 align centre middle in box 5.6 x 3.1 at (0.05, -2.8) x (0, 1) y (-1, 0) spacing 1 kerned
  constraint coincident L1.end
  constraint coincident L0.start
extrude "Extrude31" add sketch "Sketch17" along normal blind 0.001 text T0
named bodies: "3V"
